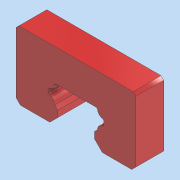
# Autodesk Inventor part: HGR20C
Saved by Autodesk Inventor 2021 (Build 250183000, 183)
## iProperties
Created: 2021-09-26
Part Number: HGR20C
Material: Generic
Document SubType Name: Modeling
Designer: 41601100
Density: 1 g/cm^3
Appearance: Default
Author: 41601100
Autodesk Inventor part; units mm, degrees
ref_plane "YZ Plane" through (0, 0, 0) normal (1, 0, 0) x (0, 1, 0)
ref_plane "XZ Plane" through (0, 0, 0) normal (0, 1, 0) x (-1, 0, 0)
ref_plane "XY Plane" through (0, 0, 0) normal (0, 0, 1) x (1, 0, 0)
sketch "Sketch1" plane through (0, 0, 0) normal (0, 0, 1) x (1, 0, 0)
  line L0 (20.5165, 15) -> (21.5, 14.0165)
  line L1 (-20.5165, 15) -> (20.5165, 15)
  line L2 (-21.5, 14.0165) -> (-20.5165, 15)
  line L3 (-21.5, -8) -> (-21.5, 14.0165)
  line L4 (-20, -9.5) -> (-21.5, -8)
  line L5 (-9.45, -9.5) -> (-20, -9.5)
  line L6 (-6.6, -6.65) -> (-9.45, -9.5)
  line L7 (-6.6, -4.35) -> (-6.6, -6.65)
  line L8 (-7.7, -3.25) -> (-6.6, -4.35)
  arc A0 (-7.7, -3.25) -> (-9.6, -1.075) centre (-9.8292, -3.1926) ccw
  line L9 (-10, -0.675) -> (-9.6, -1.075)
  line L10 (-10, 0.675) -> (-10, -0.675)
  line L11 (-9.6, 1.075) -> (-10, 0.675)
  arc A1 (-9.6, 1.075) -> (-7.7, 3.1) centre (-9.828, 3.1928) ccw
  line L12 (-7.3, 3.5) -> (-7.7, 3.1)
  line L13 (7.3, 3.5) -> (-7.3, 3.5)
  line L14 (7.7, 3.1) -> (7.3, 3.5)
  arc A2 (7.7, 3.1) -> (9.6, 1.075) centre (9.828, 3.1928) ccw
  line L15 (10, 0.675) -> (9.6, 1.075)
  line L16 (10, -0.675) -> (10, 0.675)
  line L17 (9.6, -1.075) -> (10, -0.675)
  arc A3 (9.6, -1.075) -> (7.7, -3.25) centre (9.8292, -3.1926) ccw
  line L18 (6.6, -4.35) -> (7.7, -3.25)
  line L19 (6.6, -6.65) -> (6.6, -4.35)
  line L20 (9.45, -9.5) -> (6.6, -6.65)
  line L21 (20, -9.5) -> (9.45, -9.5)
  line L22 (21.5, -8) -> (20, -9.5)
  line L23 (21.5, 14.0165) -> (21.5, -8)
  circle A4 centre (-18.75, 2.9) radius 2.625
  circle A5 centre (18.75, 2.9) radius 2.625
  point P0 (0, 0)
  point P1 (0, 0)
  constraints: 48 end point, 8 point on circle, 6 centre point
extrude "Extrusion1" add sketch "Sketch1" along normal blind 10 contours L0 L23 L22 L21 L20 L19 L18 A3 L17 L16 L15 A2 L14 L13 L12 A1 L11 L10 L9 A0 L8 L7 L6 L5 L4 L3 L2 L1 | A4 | A5
extrude "Extrusion2" cut sketch "Sketch1" along normal blind 2.1 contours A4 | A5
sketch "Sketch2" plane through (0, 0, 0) normal (0, 0, -1) x (-1, 0, 0)
  circle A0 centre (18.75, 2.9) radius 2.625 projected
  circle A1 centre (-18.75, 2.9) radius 2.625 projected
  line L0 (-7.7, -3.25) -> (-6.6, -4.35) projected
  arc A2 (-7.7, -3.25) -> (-9.6, -1.075) centre (-9.8292, -3.1926) ccw projected
  line L1 (-10, -0.675) -> (-9.6, -1.075) projected
  line L2 (-10, 0.675) -> (-10, -0.675) projected
  line L3 (-9.6, 1.075) -> (-10, 0.675) projected
  arc A3 (-9.6, 1.075) -> (-7.7, 3.1) centre (-9.828, 3.1928) ccw projected
  line L4 (-7.3, 3.5) -> (-7.7, 3.1) projected
  line L5 (7.3, 3.5) -> (-7.3, 3.5) projected
  line L6 (7.7, 3.1) -> (7.3, 3.5) projected
  arc A4 (7.7, 3.1) -> (9.6, 1.075) centre (9.828, 3.1928) ccw projected
  line L7 (10, 0.675) -> (9.6, 1.075) projected
  line L8 (10, -0.675) -> (10, 0.675) projected
  line L9 (9.6, -1.075) -> (10, -0.675) projected
  arc A5 (9.6, -1.075) -> (7.7, -3.25) centre (9.8292, -3.1926) ccw projected
  line L10 (6.6, -4.35) -> (7.7, -3.25) projected
  line L11 (6.6, -6.65) -> (6.6, -4.35) projected
  line L12 (9.45, -9.5) -> (6.6, -6.65) projected
  line L13 (20, -9.5) -> (9.45, -9.5) projected
  line L14 (21.5, -8) -> (20, -9.5) projected
  line L15 (21.5, 14.0165) -> (21.5, -8) projected
  line L16 (20.5165, 15) -> (21.5, 14.0165) projected
  line L17 (-20.5165, 15) -> (20.5165, 15) projected
  line L18 (-21.5, 14.0165) -> (-20.5165, 15) projected
  line L19 (-21.5, -8) -> (-21.5, 14.0165) projected
  line L20 (-20, -9.5) -> (-21.5, -8) projected
  line L21 (-9.45, -9.5) -> (-20, -9.5) projected
  line L22 (-6.6, -6.65) -> (-9.45, -9.5) projected
  line L23 (-6.6, -4.35) -> (-6.6, -6.65) projected
  circle A6 centre (0, 11) radius 3
  point P0 (0, 0)
  point P1 (0, 0)
  constraints: 1 centre point
extrude "Extrusion3" cut sketch "Sketch2" against normal blind 4 contours A6
body "Solid1"
